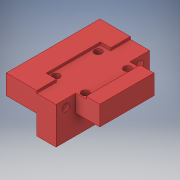
# Autodesk Inventor part: КВ33.044.502 - Фиксатор оси Y
Saved by Autodesk Inventor 2019 (Build 230136000, 136)
## iProperties
Created: 2019-08-02
Part Number: КВ33.044.502 - Фиксатор оси Y
Material: Пластик АБС
Document SubType Name: Modeling
Designer: Петров Иван
Density: 1.06 g/cm^3
Appearance: Гладкий — красный
Author: Петров Иван
Autodesk Inventor part; units mm, degrees
ref_plane "YZ Plane" through (0, 0, 0) normal (1, 0, 0) x (0, 1, 0)
ref_plane "XZ Plane" through (0, 0, 0) normal (0, 1, 0) x (-1, 0, 0)
ref_plane "XY Plane" through (0, 0, 0) normal (0, 0, 1) x (1, 0, 0)
sketch "Эскиз1" plane through (0, 0, 0) normal (1, 0, 0) x (0, 1, 0)
  line L0 (-4, 19) -> (4, 19)
  line L1 (4, 19) -> (4, -19)
  line L2 (4, -19) -> (-4, -19)
  line L3 (-4, -19) -> (-4, 19)
  line L4 (-4, 19) -> (4, -19) construction
  line L5 (4, 19) -> (-4, -19) construction
  point P0 (0, 0)
  dimension "d0" = 8
  dimension "d1" = 38
  constraints: 12 end point, 2 midpoint, 2 parallel, 1 horizontal, 1 perpendicular
  measures "d0" distance of L1.end L2.end
  measures "d1" distance of L0.end L1.end
extrude "Выдавливание1" add sketch "Эскиз1" along normal blind 20.2
sketch "Эскиз2" plane through (0, 0, 0) normal (-1, 0, 0) x (0, 0, 1)
  line L0 (0, 0) -> (-15, 0)
  line L1 (0, 0) -> (15, 0) construction
  line L2 (-15, 0) -> (15, 0)
  circle A0 centre (-15, 0) radius 1.5
  circle A1 centre (15, 0) radius 1.5
  dimension "d4" = 15
  dimension "d5" = 180
  dimension "d6" = 30
  dimension "d7" = 3
  dimension "d8" = 3
  constraints: 6 end point, 2 centre point, 2 coincident, 2 horizontal, 1 collinear, 1 point on line
  measures "d4" distance of L0.start L0.end
  measures "d5" angle of L0 L1
  measures "d6" distance of L0.end L2.end
  measures "d7" diameter of A0
  measures "d8" diameter of A1
extrude "Выдавливание2" cut sketch "Эскиз2" against normal through all
sketch "Эскиз3" plane through (0, -4, -19) normal (0, -1, 0) x (1, 0, 0)
  line L0 (0, 38) -> (20.2, 38) projected
  line L1 (0, 0) -> (20.2, 0) projected
  line L2 (20.2, 38) -> (12.4, 38)
  line L3 (12.4, 38) -> (12.4, 0)
  line L4 (12.4, 0) -> (20.2, 0)
  line L5 (20.2, 0) -> (20.2, 38)
  point P0 (0, 19)
  dimension "d11" = 7.8
  constraints: 8 end point, 2 parallel, 1 horizontal, 1 perpendicular, 1 point on line
  measures "d11" distance of L4.end L3.end
extrude "Выдавливание3" add sketch "Эскиз3" along normal blind 8
sketch "Эскиз4" plane through (20.2, 0, 0) normal (1, 0, 0) x (0, 0, -1)
  line L0 (19, -4) -> (-19, -4) projected
  line L1 (-18.1844, -4) -> (0, -4)
  line L2 (19, 4) -> (-19, 4) projected
  line L3 (-11, -4) -> (11, -4)
  line L4 (11, -4) -> (11, 4)
  line L5 (11, 4) -> (-11, 4)
  line L6 (-11, 4) -> (-11, -4)
  line L7 (-11, -4) -> (11, 4) construction
  line L8 (11, -4) -> (-11, 4) construction
  point P0 (0, 0)
  dimension "d17" = 22
  constraints: 14 end point, 3 midpoint, 2 parallel, 2 point on line, 1 horizontal, 1 perpendicular
  measures "d17" distance of L5.end L4.end
extrude "Выдавливание4" add sketch "Эскиз4" along normal blind 9.8
sketch "Эскиз5" plane through (0, 4, 19) normal (0, 1, 0) x (1, 0, 0)
  line L0 (0, 38) -> (12.4, 38) projected
  line L1 (12.4, 38) -> (24.4, 38)
  line L2 (24.4, 38) -> (24.4, 0)
  line L3 (24.4, 0) -> (12.4, 0)
  line L4 (12.4, 0) -> (12.4, 38)
  line L5 (20.2, 8) -> (30, 8) projected
  line L6 (20.2, 38) -> (20.2, 0) projected
  line L7 (24.4, 8) -> (20.2, 8)
  line L8 (20.2, 8) -> (20.2, 30)
  line L9 (20.2, 30) -> (24.4, 30)
  line L10 (24.4, 30) -> (24.4, 8)
  line L11 (12.4, 0) -> (12.4, 38) projected
  line L12 (12.4, 8) -> (8.2, 8)
  line L13 (8.2, 8) -> (8.2, 30)
  line L14 (8.2, 30) -> (12.4, 30)
  line L15 (12.4, 30) -> (12.4, 8)
  point P0 (0, 19)
  dimension "d20" = 12
  dimension "d21" = 38
  dimension "d24" = 22
  dimension "d25" = 4.2
  dimension "d26" = 4.2
  constraints: 24 end point, 6 parallel, 4 point on line, 3 horizontal, 3 perpendicular
  measures "d20" distance of L2.end L3.end
  measures "d21" distance of L1.end L2.end
  measures "d24" distance of L7.end L8.end
  measures "d25" distance of L8.end L9.end
  measures "d26" distance of L13.end L14.end
extrude "Выдавливание5" cut sketch "Эскиз5" against normal blind 1
sketch "Эскиз6" plane through (0, 3, 19) normal (0, 1, 0) x (1, 0, 0)
  circle A0 centre (10.1672, 27.1433) radius 1.5
  circle A1 centre (10.1672, 10.008) radius 1.5
  circle A2 centre (22.0732, 27.1433) radius 1.5
  circle A3 centre (22.0732, 10.008) radius 1.5
  point P0 (0, 19)
  dimension "d27" = 3
  dimension "d28" = 3
  dimension "d29" = 3
  dimension "d30" = 3
  constraints: 4 centre point
  measures "d27" diameter of A0
  measures "d28" diameter of A1
  measures "d29" diameter of A2
  measures "d30" diameter of A3
extrude "Выдавливание6" cut sketch "Эскиз6" against normal blind 4.5
sketch "Эскиз7" plane through (0, 3, 19) normal (0, 1, 0) x (1, 0, 0)
  circle A0 centre (22.0732, 27.1433) radius 1.5 projected
  circle A1 centre (10.1672, 27.1433) radius 1.5 projected
  circle A2 centre (10.1672, 10.008) radius 1.5 projected
  circle A3 centre (22.0732, 10.008) radius 1.5 projected
  line L0 (20.2, 8) -> (20.2, 0) projected
  line L1 (24.4, 8) -> (20.2, 8) projected
  line L2 (24.4, 30) -> (24.4, 8) projected
  line L3 (20.2, 30) -> (24.4, 30) projected
  line L4 (20.2, 38) -> (20.2, 30) projected
  line L5 (12.4, 38) -> (20.2, 38) projected
  line L6 (12.4, 30) -> (12.4, 38) projected
  line L7 (8.2, 30) -> (12.4, 30) projected
  line L8 (8.2, 8) -> (8.2, 30) projected
  line L9 (12.4, 8) -> (8.2, 8) projected
  line L10 (12.4, 0) -> (12.4, 8) projected
  line L11 (20.2, 0) -> (12.4, 0) projected
  point P0 (0, 19)
